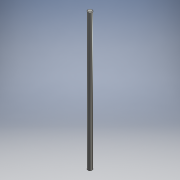
# Autodesk Inventor part: Linear rail - Y
Saved by Autodesk Inventor 2016 (Build 200138000, 138)
## iProperties
Created: 2016-12-24
Part Number: Linear rail - Y
Material: Steel, Mild
Document SubType Name: Modeling
Designer: Scott
Mass: 246.615 g
Surface Area: 127.235 cm^2
Volume: 31.4159 cm^3
Density: 7.85 g/cm^3
Appearance: Chrome - Polished Black
Author: Scott
Autodesk Inventor part; units mm, degrees
ref_plane "YZ Plane" through (0, 0, 0) normal (1, 0, 0) x (0, 1, 0)
ref_plane "XZ Plane" through (0, 0, 0) normal (0, 1, 0) x (-1, 0, 0)
ref_plane "XY Plane" through (0, 0, 0) normal (0, 0, 1) x (1, 0, 0)
sketch "Sketch1" plane through (0, 0, 0) normal (0, 0, 1) x (1, 0, 0)
  circle A0 centre (0, 0) radius 5
  dimension "d0" = 10
  constraints: 1 centre point, 1 coincident
  measures "d0" diameter of A0
extrude "Extrusion1" add sketch "Sketch1" along normal blind 320
chamfer "Chamfer1" distance 1 angle 45 2 edges at (-5, 0, 320) (-5, 0, 0)
equation "\"d1\" = frame_depth - 2 * extrusion_size"
equation "\"platform_width\" = 214"
equation "\"platform_depth\" = 214"
equation "\"bed_cl_y_offset\" = 173.25"
equation "\"frame_depth\" = 380"
equation "\"extrusion_size\" = 30"
body "Solid1"
